Autodesk Inventor part; units mm, degrees
(part 2 of 3)
  spline S192 degree 2 poles (69.3995, 110.7069) (69.4696, 110.764) (69.7263, 110.8625) (69.8923, 110.8625) knots 0 0 0 1 2 2 2
  spline S193 degree 2 poles (69.8923, 110.8625) (70.0453, 110.8625) (70.2632, 110.7614) (70.4006, 110.5669) (70.4655, 110.2945) (70.4655, 110.126) knots 0 0 0 1 2 3 4 4 4
  line L261 (70.4655, 110.126) -> (70.4655, 108.6191)
  line L262 (70.4655, 108.6191) -> (70.0842, 108.6191)
  line L263 (70.0842, 108.6191) -> (70.0842, 110.1052)
  spline S194 degree 2 poles (70.0842, 110.1052) (70.0842, 110.2141) (70.0531, 110.3775) (69.9805, 110.4865) (69.856, 110.5409) (69.7626, 110.5409) knots 0 0 0 1 2 3 4 4 4
  spline S195 degree 2 poles (69.7626, 110.5409) (69.7056, 110.5409) (69.5785, 110.502) (69.4488, 110.4346) (69.3269, 110.349) (69.2725, 110.3049) knots 0 0 0 1 2 3 4 4 4
  spline S196 degree 2 poles (69.2725, 110.3049) (69.2776, 110.2453) (69.2802, 110.1675) (69.2802, 110.1052) knots 0 0 0 1 2 2 2
  line L264 (69.2802, 110.1052) -> (69.2802, 108.6191)
  line L265 (69.2802, 108.6191) -> (68.899, 108.6191)
  line L266 (68.899, 108.6191) -> (68.899, 110.1052)
  spline S197 degree 2 poles (68.899, 110.1052) (68.899, 110.3231) (68.7538, 110.5409) (68.567, 110.5409) knots 0 0 0 1 2 2 2
  spline S198 degree 2 poles (68.567, 110.5409) (68.5074, 110.5409) (68.3699, 110.5046) (68.2376, 110.4398) (68.108, 110.3594) (68.0561, 110.3153) knots 0 0 0 1 2 3 4 4 4
  line L267 (68.0561, 110.3153) -> (68.0561, 108.6191)
  spline S199 degree 2 poles (73.6192, 110.4657) (73.5829, 110.4839) (73.4818, 110.5202) (73.3728, 110.5487) (73.2639, 110.5643) (73.2146, 110.5643) knots 0 0 0 1 2 3 4 4 4
  spline S200 degree 2 poles (73.2146, 110.5643) (73.002, 110.5643) (72.8256, 110.4372) (72.8256, 110.3101) knots 0 0 0 1 2 2 2
  spline S201 degree 2 poles (72.8256, 110.3101) (72.8256, 110.2271) (72.9423, 110.1156) (73.1265, 110.0274) (73.3521, 109.9496) (73.461, 109.8951) knots 0 0 0 1 2 3 4 4 4
  spline S202 degree 2 poles (73.461, 109.8951) (73.5388, 109.8562) (73.6996, 109.7525) (73.8267, 109.6124) (73.9071, 109.4361) (73.9071, 109.3246) knots 0 0 0 1 2 3 4 4 4
  spline S203 degree 2 poles (73.9071, 109.3246) (73.9071, 109.1223) (73.7697, 108.8396) (73.5362, 108.6658) (73.2224, 108.5854) (73.0435, 108.5854) knots 0 0 0 1 2 3 4 4 4
  spline S204 degree 2 poles (73.0435, 108.5854) (72.9734, 108.5854) (72.8023, 108.6113) (72.6285, 108.658) (72.4729, 108.7229) (72.421, 108.7592) knots 0 0 0 1 2 3 4 4 4
  line L268 (72.421, 108.7592) -> (72.5533, 109.0237)
  spline S205 degree 2 poles (72.5533, 109.0237) (72.6026, 109.0004) (72.7348, 108.9563) (72.8749, 108.9252) (73.0123, 108.907) (73.0668, 108.907) knots 0 0 0 1 2 3 4 4 4
  spline S206 degree 2 poles (73.0668, 108.907) (73.1602, 108.907) (73.3313, 108.9459) (73.461, 109.0289) (73.5388, 109.1638) (73.5388, 109.2623) knots 0 0 0 1 2 3 4 4 4
  spline S207 degree 2 poles (73.5388, 109.2623) (73.5388, 109.3375) (73.4766, 109.449) (73.3703, 109.5346) (73.2302, 109.6073) (73.072, 109.6747) (72.9086, 109.7447) (72.8334, 109.7862) knots 0 0 0 1 2 3 4 5 6 6 6
  spline S208 degree 2 poles (72.8334, 109.7862) (72.7634, 109.8277) (72.6337, 109.9237) (72.5325, 110.043) (72.4729, 110.1934) (72.4729, 110.2894) knots 0 0 0 1 2 3 4 4 4
  spline S209 degree 2 poles (72.4729, 110.2894) (72.4729, 110.4424) (72.5818, 110.6628) (72.7789, 110.7977) (73.0538, 110.8625) (73.2198, 110.8625) knots 0 0 0 1 2 3 4 4 4
  spline S210 degree 2 poles (73.2198, 110.8625) (73.2976, 110.8625) (73.4455, 110.8392) (73.5829, 110.8003) (73.6944, 110.7484) (73.7333, 110.7225) knots 0 0 0 1 2 3 4 4 4
  line L269 (73.7333, 110.7225) -> (73.6192, 110.4657)
  line L270 (75.7252, 110.8288) -> (76.1064, 110.8677)
  line L271 (76.1064, 110.8677) -> (76.1064, 108.6191)
  line L272 (76.1064, 108.6191) -> (75.7252, 108.6191)
  line L273 (75.7252, 108.6191) -> (75.7252, 108.9459)
  line L274 (75.7252, 108.9459) -> (75.6033, 108.7332)
  spline S211 degree 2 poles (75.6033, 108.7332) (75.567, 108.7073) (75.4684, 108.6554) (75.3439, 108.6139) (75.1961, 108.5854) (75.1131, 108.5854) knots 0 0 0 1 2 3 4 4 4
  spline S212 degree 2 poles (75.1131, 108.5854) (74.9523, 108.5854) (74.7215, 108.7021) (74.5737, 108.9096) (74.501, 109.1975) (74.501, 109.3661) knots 0 0 0 1 2 3 4 4 4
  line L275 (74.501, 109.3661) -> (74.501, 110.8288)
  line L276 (74.501, 110.8288) -> (74.8823, 110.8677)
  line L277 (74.8823, 110.8677) -> (74.8823, 109.3661)
  spline S213 degree 2 poles (74.8823, 109.3661) (74.8823, 109.1508) (75.056, 108.907) (75.2428, 108.907) knots 0 0 0 1 2 2 2
  spline S214 degree 2 poles (75.2428, 108.907) (75.3128, 108.907) (75.4451, 108.9511) (75.5696, 109.0185) (75.6785, 109.0989) (75.7252, 109.1378) knots 0 0 0 1 2 3 4 4 4
  line L278 (75.7252, 109.1378) -> (75.7252, 110.8288)
  spline S215 degree 2 poles (77.8571, 110.5228) (77.7767, 110.5228) (77.6185, 110.4579) (77.4732, 110.349) (77.3461, 110.2064) (77.2917, 110.126) knots 0 0 0 1 2 3 4 4 4
  line L279 (77.2917, 110.126) -> (77.2917, 108.6191)
  line L280 (77.2917, 108.6191) -> (76.9104, 108.6191)
  line L281 (76.9104, 108.6191) -> (76.9104, 110.8288)
  line L282 (76.9104, 110.8288) -> (77.2917, 110.8677)
  line L283 (77.2917, 110.8677) -> (77.2917, 110.4164)
  line L284 (77.2917, 110.4164) -> (77.4914, 110.7692)
  spline S216 degree 2 poles (77.4914, 110.7692) (77.5173, 110.7847) (77.5977, 110.8184) (77.6963, 110.8444) (77.8104, 110.8625) (77.8726, 110.8625) knots 0 0 0 1 2 3 4 4 4
  spline S217 degree 2 poles (77.8726, 110.8625) (77.9634, 110.8625) (78.0853, 110.8314) (78.1138, 110.8158) knots 0 0 0 1 2 2 2
  line L285 (78.1138, 110.8158) -> (78.0957, 110.4839)
  spline S218 degree 2 poles (78.0957, 110.4839) (78.0646, 110.4916) (77.9453, 110.5228) (77.8571, 110.5228) knots 0 0 0 1 2 2 2
  line L286 (78.215, 110.8262) -> (78.5158, 110.8262)
  line L287 (78.5158, 110.8262) -> (78.5158, 111.1374)
  spline S219 degree 2 poles (78.5158, 111.1374) (78.5158, 111.3086) (78.591, 111.5757) (78.7492, 111.7625) (79.0008, 111.8636) (79.1772, 111.8636) knots 0 0 0 1 2 3 4 4 4
  spline S220 degree 2 poles (79.1772, 111.8636) (79.268, 111.8636) (79.4184, 111.8325) (79.5455, 111.7858) (79.6518, 111.721) (79.6933, 111.6873) knots 0 0 0 1 2 3 4 4 4
  line L288 (79.6933, 111.6873) -> (79.5221, 111.4487)
  spline S221 degree 2 poles (79.5221, 111.4487) (79.4806, 111.4798) (79.3328, 111.542) (79.242, 111.542) knots 0 0 0 1 2 2 2
  spline S222 degree 2 poles (79.242, 111.542) (79.0683, 111.542) (78.8867, 111.3475) (78.8867, 111.1167) knots 0 0 0 1 2 2 2
  line L289 (78.8867, 111.1167) -> (78.8867, 110.8262)
  line L290 (78.8867, 110.8262) -> (79.4703, 110.8262)
  line L291 (79.4703, 110.8262) -> (79.4288, 110.5046)
  line L292 (79.4288, 110.5046) -> (78.8971, 110.5046)
  line L293 (78.8971, 110.5046) -> (78.8971, 108.6191)
  line L294 (78.8971, 108.6191) -> (78.5158, 108.6191)
  line L295 (78.5158, 108.6191) -> (78.5158, 110.5046)
  line L296 (78.5158, 110.5046) -> (78.215, 110.5046)
  line L297 (78.215, 110.5046) -> (78.215, 110.8262)
  line L298 (81.5658, 108.6191) -> (81.1457, 108.6191)
  line L299 (81.1457, 108.6191) -> (81.1457, 108.9433)
  line L300 (81.1457, 108.9433) -> (80.9563, 108.7203)
  spline S223 degree 2 poles (80.9563, 108.7203) (80.9226, 108.6943) (80.8345, 108.6451) (80.7437, 108.6061) (80.6529, 108.5854) (80.614, 108.5854) knots 0 0 0 1 2 3 4 4 4
  spline S224 degree 2 poles (80.614, 108.5854) (80.4636, 108.5854) (80.1887, 108.6788) (79.9812, 108.8629) (79.8593, 109.1326) (79.8593, 109.3116) knots 0 0 0 1 2 3 4 4 4
  spline S225 degree 2 poles (79.8593, 109.3116) (79.8593, 109.4983) (80.0097, 109.7732) (80.2457, 109.9548) (80.5336, 110.0456) (80.6737, 110.0456) knots 0 0 0 1 2 3 4 4 4
  spline S226 degree 2 poles (80.6737, 110.0456) (80.7878, 110.0456) (80.9615, 110.0222) (81.0238, 110.0067) knots 0 0 0 1 2 2 2
  spline S227 degree 2 poles (81.0238, 110.0067) (81.0938, 109.9885) (81.1457, 109.9652) knots 0 0 0 1 1 1
  line L301 (81.1457, 109.9652) -> (81.1457, 110.0352)
  spline S228 degree 2 poles (81.1457, 110.0352) (81.1457, 110.1545) (81.1171, 110.3412) (81.0316, 110.4735) (80.8682, 110.5409) (80.7333, 110.5409) knots 0 0 0 1 2 3 4 4 4
  spline S229 degree 2 poles (80.7333, 110.5409) (80.6244, 110.5409) (80.4247, 110.5098) (80.3469, 110.4916) knots 0 0 0 1 2 2 2
  spline S230 degree 2 poles (80.3469, 110.4916) (80.2535, 110.4709) (80.1757, 110.4476) knots 0 0 0 1 1 1
  line L302 (80.1757, 110.4476) -> (80.0305, 110.7147)
  spline S231 degree 2 poles (80.0305, 110.7147) (80.1186, 110.7562) (80.2302, 110.7873) knots 0 0 0 1 1 1
  spline S232 degree 2 poles (80.2302, 110.7873) (80.3261, 110.8158) (80.5933, 110.8625) (80.7541, 110.8625) knots 0 0 0 1 2 2 2
  spline S233 degree 2 poles (80.7541, 110.8625) (80.9849, 110.8625) (81.2857, 110.738) (81.4595, 110.5124) (81.5269, 110.1986) (81.5269, 110.0041) knots 0 0 0 1 2 3 4 4 4
  line L303 (81.5269, 110.0041) -> (81.5269, 108.9796)
  line L304 (81.5269, 108.9796) -> (81.5658, 108.6191)
  spline S234 degree 2 poles (81.1457, 109.6902) (81.0886, 109.698) (81.0238, 109.7058) knots 0 0 0 1 1 1
  spline S235 degree 2 poles (81.0238, 109.7058) (80.9719, 109.711) (80.8293, 109.724) (80.7541, 109.724) knots 0 0 0 1 2 2 2
  spline S236 degree 2 poles (80.7541, 109.724) (80.6399, 109.724) (80.4532, 109.6799) (80.3157, 109.5813) (80.2405, 109.4257) (80.2405, 109.3116) knots 0 0 0 1 2 3 4 4 4
  spline S237 degree 2 poles (80.2405, 109.3116) (80.2405, 109.2234) (80.3002, 109.073) (80.4065, 108.9641) (80.5492, 108.907) (80.6296, 108.907) knots 0 0 0 1 2 3 4 4 4
  spline S238 degree 2 poles (80.6296, 108.907) (80.6685, 108.907) (80.7566, 108.9303) (80.8422, 108.9641) (80.9278, 109.0133) (80.9667, 109.0367) knots 0 0 0 1 2 3 4 4 4
  spline S239 degree 2 poles (80.9667, 109.0367) (81.0575, 109.0963) (81.1457, 109.1689) knots 0 0 0 1 1 1
  line L305 (81.1457, 109.1689) -> (81.1457, 109.6902)
  spline S240 degree 2 poles (83.4461, 110.3827) (83.3683, 110.4527) (83.1531, 110.5409) (83.039, 110.5409) knots 0 0 0 1 2 2 2
  spline S241 degree 2 poles (83.039, 110.5409) (82.8704, 110.5409) (82.6344, 110.4138) (82.4865, 110.1986) (82.4191, 109.9107) (82.4191, 109.7525) knots 0 0 0 1 2 3 4 4 4
  spline S242 degree 2 poles (82.4191, 109.7525) (82.4191, 109.5865) (82.4813, 109.2882) (82.6292, 109.06) (82.8756, 108.9252) (83.0623, 108.9252) knots 0 0 0 1 2 3 4 4 4
  spline S243 degree 2 poles (83.0623, 108.9252) (83.2153, 108.9252) (83.4306, 108.9978) (83.4902, 109.0367) knots 0 0 0 1 2 2 2
  line L306 (83.4902, 109.0367) -> (83.6329, 108.754)
  spline S244 degree 2 poles (83.6329, 108.754) (83.5214, 108.6788) (83.2231, 108.5854) (83.0338, 108.5854) knots 0 0 0 1 2 2 2
  spline S245 degree 2 poles (83.0338, 108.5854) (82.7822, 108.5854) (82.4061, 108.7851) (82.1546, 109.1145) (82.0275, 109.5476) (82.0275, 109.7784) knots 0 0 0 1 2 3 4 4 4
  spline S246 degree 2 poles (82.0275, 109.7784) (82.0275, 109.9859) (82.1494, 110.3775) (82.4009, 110.681) (82.7848, 110.8625) (83.0441, 110.8625) knots 0 0 0 1 2 3 4 4 4
  spline S247 degree 2 poles (83.0441, 110.8625) (83.2283, 110.8625) (83.5188, 110.7484) (83.6458, 110.6084) knots 0 0 0 1 2 2 2
  line L307 (83.6458, 110.6084) -> (83.4461, 110.3827)
  spline S248 degree 2 poles (85.7725, 108.8785) (85.7103, 108.8136) (85.5625, 108.7073) (85.3809, 108.6269) (85.1631, 108.5854) (85.0282, 108.5854) knots 0 0 0 1 2 3 4 4 4
  spline S249 degree 2 poles (85.0282, 108.5854) (84.7611, 108.5854) (84.385, 108.7747) (84.1464, 109.0911) (84.0349, 109.5009) (84.0349, 109.724) knots 0 0 0 1 2 3 4 4 4
  spline S250 degree 2 poles (84.0349, 109.724) (84.0349, 109.8666) (84.0867, 110.1467) (84.1905, 110.3983) (84.3487, 110.6161) (84.5562, 110.7718) (84.8207, 110.8625) (84.9789, 110.8625) knots 0 0 0 1 2 3 4 5 6 6 6
  spline S251 degree 2 poles (84.9789, 110.8625) (85.1942, 110.8625) (85.5132, 110.7225) (85.7207, 110.4683) (85.8218, 110.1156) (85.8218, 109.9003) knots 0 0 0 1 2 3 4 4 4
  spline S252 degree 2 poles (85.8218, 109.9003) (85.8218, 109.8381) (85.814, 109.6902) (85.8063, 109.6228) knots 0 0 0 1 2 2 2
  line L308 (85.8063, 109.6228) -> (84.4161, 109.6228)
  spline S253 degree 2 poles (84.4161, 109.6228) (84.4161, 109.4724) (84.4991, 109.213) (84.647, 109.0185) (84.857, 108.907) (84.9893, 108.907) knots 0 0 0 1 2 3 4 4 4
  spline S254 degree 2 poles (84.9893, 108.907) (85.1164, 108.907) (85.3083, 108.9459) (85.4432, 109.0004) (85.5313, 109.0548) (85.5547, 109.0704) knots 0 0 0 1 2 3 4 4 4
  line L309 (85.5547, 109.0704) -> (85.7725, 108.8785)
  spline S255 degree 2 poles (85.4406, 109.9237) (85.4432, 109.947) (85.4458, 109.9911) (85.4458, 110.0118) knots 0 0 0 1 2 2 2
  spline S256 degree 2 poles (85.4458, 110.0118) (85.4458, 110.126) (85.3913, 110.3205) (85.285, 110.4631) (85.1216, 110.5435) (85.0075, 110.5435) knots 0 0 0 1 2 3 4 4 4
  spline S257 degree 2 poles (85.0075, 110.5435) (84.8752, 110.5435) (84.6833, 110.4579) (84.5536, 110.3231) (84.4732, 110.1623) (84.455, 110.0897) knots 0 0 0 1 2 3 4 4 4
  line L310 (84.455, 110.0897) -> (84.3487, 109.8692)
  line L311 (84.3487, 109.8692) -> (84.7066, 109.9237)
  line L312 (84.7066, 109.9237) -> (85.4406, 109.9237)
  spline S258 degree 2 poles (87.4454, 108.6191) (87.4454, 108.4402) (87.4091, 108.1315) (87.2872, 107.9033) (87.0486, 107.7762) (86.8437, 107.7762) knots 0 0 0 1 2 3 4 4 4
  spline S259 degree 2 poles (86.8437, 107.7762) (86.8048, 107.7762) (86.7218, 107.7814) (86.644, 107.7944) (86.5817, 107.8151) (86.5636, 107.8255) knots 0 0 0 1 2 3 4 4 4
  line L313 (86.5636, 107.8255) -> (86.7036, 108.0797)
  spline S260 degree 2 poles (86.7036, 108.0797) (86.714, 108.0745) (86.7296, 108.0719) knots 0 0 0 1 1 1
  spline S261 degree 2 poles (86.7296, 108.0719) (86.7451, 108.0719) (86.7814, 108.0693) (86.8022, 108.0693) knots 0 0 0 1 2 2 2
  spline S262 degree 2 poles (86.8022, 108.0693) (86.8904, 108.0693) (86.9889, 108.1523) (87.0356, 108.2975) (87.0434, 108.4868) (87.0434, 108.5906) knots 0 0 0 1 2 3 4 4 4
  line L314 (87.0434, 108.5906) -> (87.0434, 111.0155)
  spline S263 degree 2 poles (87.0434, 111.0155) (87.0434, 111.1193) (87.0356, 111.3086) (86.9889, 111.4539) (86.8904, 111.5368) (86.8022, 111.5368) knots 0 0 0 1 2 3 4 4 4
  spline S264 degree 2 poles (86.8022, 111.5368) (86.7814, 111.5368) (86.7451, 111.5343) (86.7296, 111.5317) knots 0 0 0 1 2 2 2
  spline S265 degree 2 poles (86.7296, 111.5317) (86.714, 111.5291) (86.7036, 111.5291) knots 0 0 0 1 1 1
  line L315 (86.7036, 111.5291) -> (86.5636, 111.7806)
  spline S266 degree 2 poles (86.5636, 111.7806) (86.5817, 111.7936) (86.644, 111.8118) (86.7218, 111.8247) (86.8048, 111.8299) (86.8437, 111.8299) knots 0 0 0 1 2 3 4 4 4
  spline S267 degree 2 poles (86.8437, 111.8299) (87.0486, 111.8299) (87.2872, 111.7028) (87.4091, 111.4746) (87.4454, 111.166) (87.4454, 110.987) knots 0 0 0 1 2 3 4 4 4
  line L316 (87.4454, 110.987) -> (87.4454, 108.6191)
  line L317 (32.347, 101.896) -> (32.347, 102.2176)
  line L318 (32.347, 102.2176) -> (32.8397, 102.2176)
  line L319 (32.8397, 102.2176) -> (32.8397, 104.1549)
  line L320 (32.8397, 104.1549) -> (32.9565, 104.6114)
  line L321 (32.9565, 104.6114) -> (32.6841, 104.2379)
  line L322 (32.6841, 104.2379) -> (32.2588, 103.8619)
  line L323 (32.2588, 103.8619) -> (32.0409, 104.1031)
  line L324 (32.0409, 104.1031) -> (32.9616, 104.946)
  line L325 (32.9616, 104.946) -> (33.2625, 104.9071)
  line L326 (33.2625, 104.9071) -> (33.2625, 102.2176)
  line L327 (33.2625, 102.2176) -> (33.7553, 102.2176)
  line L328 (33.7553, 102.2176) -> (33.7553, 101.896)
  line L329 (33.7553, 101.896) -> (32.347, 101.896)
  line L330 (34.829, 101.6963) -> (34.4062, 101.6963)
  line L331 (34.4062, 101.6963) -> (35.8327, 105.1068)
  line L332 (35.8327, 105.1068) -> (36.2321, 105.1068)
  line L333 (36.2321, 105.1068) -> (34.829, 101.6963)
  line L334 (38.6415, 102.4977) -> (38.281, 102.4977)
  line L335 (38.281, 102.4977) -> (38.281, 101.896)
  line L336 (38.281, 101.896) -> (37.8582, 101.896)
  line L337 (37.8582, 101.896) -> (37.8582, 102.4977)
  line L338 (37.8582, 102.4977) -> (36.6626, 102.4977)
  line L339 (36.6626, 102.4977) -> (36.6626, 102.84)
  line L340 (36.6626, 102.84) -> (37.6352, 104.946)
  line L341 (37.6352, 104.946) -> (38.0164, 104.9071)
  line L342 (38.0164, 104.9071) -> (37.1813, 103.0994)
  line L343 (37.1813, 103.0994) -> (36.9946, 102.8193)
  line L344 (36.9946, 102.8193) -> (37.8582, 102.8193)
  line L345 (37.8582, 102.8193) -> (37.8582, 103.6362)
  line L346 (37.8582, 103.6362) -> (38.281, 103.6025)
  line L347 (38.281, 103.6025) -> (38.281, 102.8193)
  line L348 (38.281, 102.8193) -> (38.6726, 102.8193)
  line L349 (38.6726, 102.8193) -> (38.6415, 102.4977)
  line L350 (40.3273, 104.9071) -> (40.3273, 104.7074)
  spline S268 degree 2 poles (40.3273, 104.7074) (40.3273, 104.6295) (40.2988, 104.4065) (40.2832, 104.2976) knots 0 0 0 1 2 2 2
  spline S269 degree 2 poles (40.2832, 104.2976) (40.2624, 104.1731) (40.2391, 104.0382) knots 0 0 0 1 1 1
  line L351 (40.2391, 104.0382) -> (40.0653, 104.0382)
  spline S270 degree 2 poles (40.0653, 104.0382) (40.042, 104.1731) (40.0212, 104.2976) knots 0 0 0 1 1 1
  spline S271 degree 2 poles (40.0212, 104.2976) (40.0057, 104.4065) (39.9772, 104.6295) (39.9772, 104.7074) knots 0 0 0 1 2 2 2
  line L352 (39.9772, 104.7074) -> (39.9772, 104.9071)
  line L353 (39.9772, 104.9071) -> (40.3273, 104.9071)
  line L354 (39.723, 104.9071) -> (39.723, 104.7074)
  spline S272 degree 2 poles (39.723, 104.7074) (39.723, 104.6295) (39.6945, 104.4065) (39.6789, 104.2976) knots 0 0 0 1 2 2 2
  spline S273 degree 2 poles (39.6789, 104.2976) (39.6582, 104.1731) (39.6348, 104.0382) knots 0 0 0 1 1 1
  line L355 (39.6348, 104.0382) -> (39.461, 104.0382)
  spline S274 degree 2 poles (39.461, 104.0382) (39.4377, 104.1731) (39.417, 104.2976) knots 0 0 0 1 1 1
  spline S275 degree 2 poles (39.417, 104.2976) (39.4014, 104.4065) (39.3729, 104.6295) (39.3729, 104.7074) knots 0 0 0 1 2 2 2
  line L356 (39.3729, 104.7074) -> (39.3729, 104.9071)
  line L357 (39.3729, 104.9071) -> (39.723, 104.9071)
  line L358 (42.4851, 104.7463) -> (42.4462, 105.1094)
  line L359 (42.4462, 105.1094) -> (42.8664, 105.1483)
  line L360 (42.8664, 105.1483) -> (42.8664, 103.8515)
  line L361 (42.8664, 103.8515) -> (43.0375, 104.0356)
  spline S276 degree 2 poles (43.0375, 104.0356) (43.1387, 104.0823) (43.3643, 104.1394) (43.4758, 104.1394) knots 0 0 0 1 2 2 2
  spline S277 degree 2 poles (43.4758, 104.1394) (43.6418, 104.1394) (43.9375, 104.0019) (44.1605, 103.7348) (44.2902, 103.3457) (44.2902, 103.0942) knots 0 0 0 1 2 3 4 4 4
  spline S278 degree 2 poles (44.2902, 103.0942) (44.2902, 102.8167) (44.1398, 102.3628) (43.8701, 102.0386) (43.4992, 101.8622) (43.2761, 101.8622) knots 0 0 0 1 2 3 4 4 4
  spline S279 degree 2 poles (43.2761, 101.8622) (43.1516, 101.8622) (42.9053, 101.8804) (42.6926, 101.9115) (42.5292, 101.9478) (42.4851, 101.966) knots 0 0 0 1 2 3 4 4 4
  line L362 (42.4851, 101.966) -> (42.4851, 104.7463)
  spline S280 degree 2 poles (42.8664, 102.2409) (42.9053, 102.2279) (43.0038, 102.2072) (43.1179, 102.1916) (43.2398, 102.1838) (43.2943, 102.1838) knots 0 0 0 1 2 3 4 4 4
  spline S281 degree 2 poles (43.2943, 102.1838) (43.4188, 102.1838) (43.6055, 102.2642) (43.7404, 102.3991) (43.8312, 102.5807) (43.8882, 102.7829) (43.909, 103.0008) (43.909, 103.102) knots 0 0 0 1 2 3 4 5 6 6 6
  spline S282 degree 2 poles (43.909, 103.102) (43.909, 103.3043) (43.8337, 103.5766) (43.7015, 103.7452) (43.5329, 103.8178) (43.4369, 103.8178) knots 0 0 0 1 2 3 4 4 4
  spline S283 degree 2 poles (43.4369, 103.8178) (43.2787, 103.8178) (42.9908, 103.6959) (42.8664, 103.5921) knots 0 0 0 1 2 2 2
  line L363 (42.8664, 103.5921) -> (42.8664, 102.2409)
  line L364 (45.2758, 101.896) -> (44.8945, 101.896)
  line L365 (44.8945, 101.896) -> (44.8945, 104.0149)
  line L366 (44.8945, 104.0149) -> (45.2758, 104.0564)
  line L367 (45.2758, 104.0564) -> (45.2758, 101.896)
  line L368 (44.8815, 104.9071) -> (45.2887, 104.9071)
  line L369 (45.2887, 104.9071) -> (45.2887, 104.5051)
  line L370 (45.2887, 104.5051) -> (44.8815, 104.5051)
  line L371 (44.8815, 104.5051) -> (44.8815, 104.9071)
  spline S284 degree 2 poles (46.4792, 102.6507) (46.4792, 102.5184) (46.5103, 102.3395) (46.5673, 102.2305) (46.6529, 102.1838) (46.71, 102.1838) knots 0 0 0 1 2 3 4 4 4
  spline S285 degree 2 poles (46.71, 102.1838) (46.7541, 102.1838) (46.8267, 102.1942) (46.8526, 102.202) knots 0 0 0 1 2 2 2
  spline S286 degree 2 poles (46.8526, 102.202) (46.8837, 102.2098) (46.9071, 102.2202) knots 0 0 0 1 1 1
  line L372 (46.9071, 102.2202) -> (47.0445, 101.9764)
  spline S287 degree 2 poles (47.0445, 101.9764) (47.029, 101.9608) (46.959, 101.9219) (46.863, 101.8856) (46.7411, 101.8622) (46.6711, 101.8622) knots 0 0 0 1 2 3 4 4 4
  spline S288 degree 2 poles (46.6711, 101.8622) (46.4895, 101.8622) (46.2639, 101.9945) (46.1394, 102.2227) (46.0979, 102.5262) (46.0979, 102.6974) knots 0 0 0 1 2 3 4 4 4
  line L373 (46.0979, 102.6974) -> (46.0979, 103.7815)
  line L374 (46.0979, 103.7815) -> (45.7971, 103.7815)
  line L375 (45.7971, 103.7815) -> (45.7971, 104.1031)
  line L376 (45.7971, 104.1031) -> (46.0979, 104.1031)
  line L377 (46.0979, 104.1031) -> (46.0979, 104.5232)
  line L378 (46.0979, 104.5232) -> (46.4688, 104.7463)
  line L379 (46.4688, 104.7463) -> (46.4688, 104.1031)
  line L380 (46.4688, 104.1031) -> (47.1509, 104.1031)
  line L381 (47.1509, 104.1031) -> (47.112, 103.7815)
  line L382 (47.112, 103.7815) -> (46.4792, 103.7815)
  line L383 (46.4792, 103.7815) -> (46.4792, 102.6507)
  spline S289 degree 2 poles (47.5062, 102.1631) (47.5062, 102.2202) (47.5529, 102.3265) (47.6333, 102.4043) (47.7422, 102.451) (47.8045, 102.451) knots 0 0 0 1 2 3 4 4 4
  spline S290 degree 2 poles (47.8045, 102.451) (47.8615, 102.451) (47.9678, 102.4095) (48.0508, 102.3291) (48.1001, 102.2072) (48.1001, 102.1294) knots 0 0 0 1 2 3 4 4 4
  spline S291 degree 2 poles (48.1001, 102.1294) (48.1001, 102.023) (48.0742, 101.8233) (47.9912, 101.6185) (47.8382, 101.4058) (47.7137, 101.2917) knots 0 0 0 1 2 3 4 4 4
  line L384 (47.7137, 101.2917) -> (47.6099, 101.3383)
  spline S292 degree 2 poles (47.6099, 101.3383) (47.6566, 101.4265) (47.6929, 101.5199) knots 0 0 0 1 1 1
  spline S293 degree 2 poles (47.6929, 101.5199) (47.7241, 101.5977) (47.7733, 101.7844) (47.7733, 101.8726) knots 0 0 0 1 2 2 2
  spline S294 degree 2 poles (47.7733, 101.8726) (47.7241, 101.8752) (47.6255, 101.9167) (47.5503, 101.9867) (47.5062, 102.0957) (47.5062, 102.1631) knots 0 0 0 1 2 3 4 4 4
  line L385 (51.3369, 104.1057) -> (51.7181, 104.1446)
  line L386 (51.7181, 104.1446) -> (51.7181, 101.896)
  line L387 (51.7181, 101.896) -> (51.3369, 101.896)
  line L388 (51.3369, 101.896) -> (51.3369, 102.2227)
  line L389 (51.3369, 102.2227) -> (51.215, 102.0101)
  spline S295 degree 2 poles (51.215, 102.0101) (51.1786, 101.9841) (51.0801, 101.9323) (50.9556, 101.8908) (50.8078, 101.8622) (50.7248, 101.8622) knots 0 0 0 1 2 3 4 4 4
  spline S296 degree 2 poles (50.7248, 101.8622) (50.564, 101.8622) (50.3332, 101.979) (50.1853, 102.1864) (50.1127, 102.4743) (50.1127, 102.6429) knots 0 0 0 1 2 3 4 4 4
  line L390 (50.1127, 102.6429) -> (50.1127, 104.1057)
  line L391 (50.1127, 104.1057) -> (50.494, 104.1446)
  line L392 (50.494, 104.1446) -> (50.494, 102.6429)
  spline S297 degree 2 poles (50.494, 102.6429) (50.494, 102.4276) (50.6677, 102.1838) (50.8545, 102.1838) knots 0 0 0 1 2 2 2
  spline S298 degree 2 poles (50.8545, 102.1838) (50.9245, 102.1838) (51.0568, 102.2279) (51.1812, 102.2954) (51.2902, 102.3758) (51.3369, 102.4147) knots 0 0 0 1 2 3 4 4 4
  line L393 (51.3369, 102.4147) -> (51.3369, 104.1057)
  spline S299 degree 2 poles (53.448, 103.7426) (53.4117, 103.7607) (53.3105, 103.797) (53.2016, 103.8256) (53.0927, 103.8411) (53.0434, 103.8411) knots 0 0 0 1 2 3 4 4 4
  spline S300 degree 2 poles (53.0434, 103.8411) (52.8307, 103.8411) (52.6544, 103.714) (52.6544, 103.5869) knots 0 0 0 1 2 2 2
  spline S301 degree 2 poles (52.6544, 103.5869) (52.6544, 103.504) (52.7711, 103.3924) (52.9552, 103.3043) (53.1809, 103.2264) (53.2898, 103.172) knots 0 0 0 1 2 3 4 4 4
  spline S302 degree 2 poles (53.2898, 103.172) (53.3676, 103.1331) (53.5284, 103.0293) (53.6555, 102.8893) (53.7359, 102.7129) (53.7359, 102.6014) knots 0 0 0 1 2 3 4 4 4
  spline S303 degree 2 poles (53.7359, 102.6014) (53.7359, 102.3991) (53.5984, 102.1164) (53.365, 101.9426) (53.0512, 101.8622) (52.8722, 101.8622) knots 0 0 0 1 2 3 4 4 4
  spline S304 degree 2 poles (52.8722, 101.8622) (52.8022, 101.8622) (52.631, 101.8882) (52.4573, 101.9349) (52.3016, 101.9997) (52.2498, 102.036) knots 0 0 0 1 2 3 4 4 4
  line L394 (52.2498, 102.036) -> (52.382, 102.3006)
  spline S305 degree 2 poles (52.382, 102.3006) (52.4313, 102.2772) (52.5636, 102.2331) (52.7036, 102.202) (52.8411, 102.1838) (52.8956, 102.1838) knots 0 0 0 1 2 3 4 4 4
  spline S306 degree 2 poles (52.8956, 102.1838) (52.9889, 102.1838) (53.1601, 102.2227) (53.2898, 102.3057) (53.3676, 102.4406) (53.3676, 102.5392) knots 0 0 0 1 2 3 4 4 4
  spline S307 degree 2 poles (53.3676, 102.5392) (53.3676, 102.6144) (53.3053, 102.7259) (53.199, 102.8115) (53.059, 102.8841) (52.9008, 102.9515) (52.7374, 103.0216) (52.6622, 103.0631) knots 0 0 0 1 2 3 4 5 6 6 6
  spline S308 degree 2 poles (52.6622, 103.0631) (52.5921, 103.1045) (52.4624, 103.2005) (52.3613, 103.3198) (52.3016, 103.4702) (52.3016, 103.5662) knots 0 0 0 1 2 3 4 4 4
  spline S309 degree 2 poles (52.3016, 103.5662) (52.3016, 103.7192) (52.4106, 103.9397) (52.6077, 104.0745) (52.8826, 104.1394) (53.0486, 104.1394) knots 0 0 0 1 2 3 4 4 4
  spline S310 degree 2 poles (53.0486, 104.1394) (53.1264, 104.1394) (53.2742, 104.116) (53.4117, 104.0771) (53.5232, 104.0253) (53.5621, 103.9993) knots 0 0 0 1 2 3 4 4 4
  line L395 (53.5621, 103.9993) -> (53.448, 103.7426)
  spline S311 degree 2 poles (55.8652, 102.1553) (55.8029, 102.0905) (55.6551, 101.9841) (55.4735, 101.9037) (55.2557, 101.8622) (55.1208, 101.8622) knots 0 0 0 1 2 3 4 4 4
  spline S312 degree 2 poles (55.1208, 101.8622) (54.8537, 101.8622) (54.4776, 102.0516) (54.239, 102.368) (54.1275, 102.7778) (54.1275, 103.0008) knots 0 0 0 1 2 3 4 4 4
  spline S313 degree 2 poles (54.1275, 103.0008) (54.1275, 103.1435) (54.1794, 103.4236) (54.2831, 103.6751) (54.4413, 103.893) (54.6488, 104.0486) (54.9133, 104.1394) (55.0715, 104.1394) knots 0 0 0 1 2 3 4 5 6 6 6
  spline S314 degree 2 poles (55.0715, 104.1394) (55.2868, 104.1394) (55.6058, 103.9993) (55.8133, 103.7452) (55.9144, 103.3924) (55.9144, 103.1772) knots 0 0 0 1 2 3 4 4 4
  spline S315 degree 2 poles (55.9144, 103.1772) (55.9144, 103.1149) (55.9067, 102.9671) (55.8989, 102.8997) knots 0 0 0 1 2 2 2
  line L396 (55.8989, 102.8997) -> (54.5087, 102.8997)
  spline S316 degree 2 poles (54.5087, 102.8997) (54.5087, 102.7492) (54.5917, 102.4899) (54.7396, 102.2954) (54.9497, 102.1838) (55.0819, 102.1838) knots 0 0 0 1 2 3 4 4 4
  spline S317 degree 2 poles (55.0819, 102.1838) (55.209, 102.1838) (55.4009, 102.2227) (55.5358, 102.2772) (55.624, 102.3317) (55.6473, 102.3472) knots 0 0 0 1 2 3 4 4 4
  line L397 (55.6473, 102.3472) -> (55.8652, 102.1553)
  spline S318 degree 2 poles (55.5332, 103.2005) (55.5358, 103.2239) (55.5384, 103.2679) (55.5384, 103.2887) knots 0 0 0 1 2 2 2
  spline S319 degree 2 poles (55.5384, 103.2887) (55.5384, 103.4028) (55.4839, 103.5973) (55.3776, 103.74) (55.2142, 103.8204) (55.1001, 103.8204) knots 0 0 0 1 2 3 4 4 4
  spline S320 degree 2 poles (55.1001, 103.8204) (54.9678, 103.8204) (54.7759, 103.7348) (54.6462, 103.5999) (54.5658, 103.4391) (54.5477, 103.3665) knots 0 0 0 1 2 3 4 4 4
  line L398 (54.5477, 103.3665) -> (54.4413, 103.146)
  line L399 (54.4413, 103.146) -> (54.7992, 103.2005)
  line L400 (54.7992, 103.2005) -> (55.5332, 103.2005)
  spline S321 degree 2 poles (58.7466, 101.8622) (58.5754, 101.8622) (58.2901, 101.9919) (58.0645, 102.2176) (57.8933, 102.5184) (57.7792, 102.8608) (57.7221, 103.2239) (57.7221, 103.4028) knots 0 0 0 1 2 3 4 5 6 6 6
  spline S322 degree 2 poles (57.7221, 103.4028) (57.7221, 103.5818) (57.7714, 103.9526) (57.8752, 104.2924) (58.0386, 104.5906) (58.2642, 104.8111) (58.5599, 104.9408) (58.7466, 104.9408) knots 0 0 0 1 2 3 4 5 6 6 6
  spline S323 degree 2 poles (58.7466, 104.9408) (58.9178, 104.9408) (59.2031, 104.8111) (59.4287, 104.5855) (59.5999, 104.2846) (59.714, 103.9423) (59.771, 103.5766) (59.771, 103.4028) knots 0 0 0 1 2 3 4 5 6 6 6
  spline S324 degree 2 poles (59.771, 103.4028) (59.771, 103.2213) (59.7218, 102.8504) (59.618, 102.5106) (59.4546, 102.2124) (59.229, 101.9919) (58.9307, 101.8622) (58.7466, 101.8622) knots 0 0 0 1 2 3 4 5 6 6 6
  spline S325 degree 2 poles (58.1397, 103.4884) (58.1397, 103.3717) (58.1553, 103.0916) (58.2045, 102.8089) (58.2901, 102.5443) (58.4276, 102.3369) (58.6273, 102.2124) (58.7622, 102.2124) knots 0 0 0 1 2 3 4 5 6 6 6
  spline S326 degree 2 poles (58.7622, 102.2124) (58.884, 102.2124) (59.0682, 102.3057) (59.2005, 102.4691) (59.2835, 102.6844) (59.3327, 102.9282) (59.3535, 103.1901) (59.3535, 103.3146) knots 0 0 0 1 2 3 4 5 6 6 6
  spline S327 degree 2 poles (59.3535, 103.3146) (59.3535, 103.4313) (59.3379, 103.7114) (59.2886, 103.9915) (59.2031, 104.2587) (59.0656, 104.4636) (58.8659, 104.5881) (58.731, 104.5881) knots 0 0 0 1 2 3 4 5 6 6 6
  spline S328 degree 2 poles (58.731, 104.5881) (58.6091, 104.5881) (58.425, 104.4947) (58.2927, 104.3339) (58.2097, 104.116) (58.1604, 103.8722) (58.1397, 103.6129) (58.1397, 103.4884) knots 0 0 0 1 2 3 4 5 6 6 6
  spline S329 degree 2 poles (60.3235, 102.1968) (60.3235, 102.2642) (60.3753, 102.3861) (60.4661, 102.4769) (60.5828, 102.5288) (60.6528, 102.5288) knots 0 0 0 1 2 3 4 4 4
  spline S330 degree 2 poles (60.6528, 102.5288) (60.7203, 102.5288) (60.8396, 102.4769) (60.9303, 102.3861) (60.9822, 102.2642) (60.9822, 102.1968) knots 0 0 0 1 2 3 4 4 4
  spline S331 degree 2 poles (60.9822, 102.1968) (60.9822, 102.1294) (60.9303, 102.0075) (60.8422, 101.9167) (60.7229, 101.8622) (60.6554, 101.8622) knots 0 0 0 1 2 3 4 4 4
  spline S332 degree 2 poles (60.6554, 101.8622) (60.588, 101.8622) (60.4661, 101.9167) (60.3753, 102.0075) (60.3235, 102.1294) (60.3235, 102.1968) knots 0 0 0 1 2 3 4 4 4
  line L401 (61.7862, 104.5855) -> (61.8147, 104.9071)
  line L402 (61.8147, 104.9071) -> (63.2801, 104.9071)
  line L403 (63.2801, 104.9071) -> (63.2801, 104.627)
  spline S333 degree 2 poles (63.2801, 104.627) (63.2568, 104.5466) (63.1426, 104.3702) (62.987, 104.1938) (62.8055, 104.0201) (62.7121, 103.9423) knots 0 0 0 1 2 3 4 4 4
  line L404 (62.7121, 103.9423) -> (62.4476, 103.7944)
  spline S334 degree 2 poles (62.4476, 103.7944) (62.4683, 103.797) (62.5306, 103.7996) (62.5591, 103.7996) knots 0 0 0 1 2 2 2
  spline S335 degree 2 poles (62.5591, 103.7996) (62.7536, 103.7996) (63.0882, 103.7037) (63.3346, 103.5091) (63.4772, 103.2083) (63.4772, 103.006) knots 0 0 0 1 2 3 4 4 4
  spline S336 degree 2 poles (63.4772, 103.006) (63.4772, 102.8115) (63.332, 102.4951) (63.083, 102.2487) (62.7458, 102.0697) (62.362, 101.953) (61.9522, 101.896) (61.7551, 101.896) knots 0 0 0 1 2 3 4 5 6 6 6
  line L405 (61.7551, 101.896) -> (61.7551, 102.2176)
  spline S337 degree 2 poles (61.7551, 102.2176) (61.9211, 102.2227) (62.2427, 102.272) (62.5306, 102.3576) (62.7769, 102.4821) (62.9533, 102.6507) (63.0545, 102.8582) (63.0545, 102.9878) knots 0 0 0 1 2 3 4 5 6 6 6
  spline S338 degree 2 poles (63.0545, 102.9878) (63.0545, 103.1305) (62.9326, 103.325) (62.7199, 103.4365) (62.432, 103.4832) (62.2686, 103.4832) knots 0 0 0 1 2 3 4 4 4
  spline S339 degree 2 poles (62.2686, 103.4832) (62.2038, 103.4832) (62.0533, 103.478) (61.9937, 103.4728) knots 0 0 0 1 2 2 2
  line L406 (61.9937, 103.4728) -> (61.9937, 103.7841)
  spline S340 degree 2 poles (61.9937, 103.7841) (62.0767, 103.8437) (62.2686, 103.9967) (62.4657, 104.1627) (62.6525, 104.3339) (62.8055, 104.4869) (62.9092, 104.6192) (62.9248, 104.6659) knots 0 0 0 1 2 3 4 5 6 6 6
  line L407 (62.9248, 104.6659) -> (62.6213, 104.5855)
  line L408 (62.6213, 104.5855) -> (61.7862, 104.5855)
  spline S341 degree 2 poles (65.6636, 103.2264) (65.5443, 103.1331) (65.3056, 103.0449) (65.1552, 103.0449) knots 0 0 0 1 2 2 2
  spline S342 degree 2 poles (65.1552, 103.0449) (64.9607, 103.0449) (64.6184, 103.1746) (64.3668, 103.4158) (64.2215, 103.7555) (64.2215, 103.9656) knots 0 0 0 1 2 3 4 4 4
  spline S343 degree 2 poles (64.2215, 103.9656) (64.2215, 104.1809) (64.359, 104.5388) (64.6158, 104.7981) (64.9789, 104.9408) (65.2019, 104.9408) knots 0 0 0 1 2 3 4 4 4
  spline S344 degree 2 poles (65.2019, 104.9408) (65.4042, 104.9408) (65.7102, 104.8163) (65.9359, 104.6114) (66.0863, 104.3469) (66.1745, 104.0616) (66.2134, 103.7815) (66.2134, 103.6622) knots 0 0 0 1 2 3 4 5 6 6 6
  spline S345 degree 2 poles (66.2134, 103.6622) (66.2134, 103.4287) (66.12, 102.9852) (65.9359, 102.5936) (65.6713, 102.2616) (65.3342, 102.0179) (64.9218, 101.8726) (64.6884, 101.8622) knots 0 0 0 1 2 3 4 5 6 6 6
  line L409 (64.6884, 101.8622) -> (64.6261, 102.1968)
  spline S346 degree 2 poles (64.6261, 102.1968) (64.8673, 102.2098) (65.2901, 102.4147) (65.6117, 102.7518) (65.8114, 103.2057) (65.8244, 103.4625) knots 0 0 0 1 2 3 4 4 4
  line L410 (65.8244, 103.4625) -> (65.6636, 103.2264)
  spline S347 degree 2 poles (65.801, 103.8074) (65.7958, 103.9578) (65.718, 104.2405) (65.578, 104.4636) (65.3627, 104.5984) (65.2201, 104.5984) knots 0 0 0 1 2 3 4 4 4
  spline S348 degree 2 poles (65.2201, 104.5984) (65.0826, 104.5984) (64.8673, 104.5102) (64.7143, 104.3546) (64.6313, 104.1342) (64.6313, 104.0019) knots 0 0 0 1 2 3 4 4 4
  spline S349 degree 2 poles (64.6313, 104.0019) (64.6313, 103.8696) (64.6988, 103.6466) (64.831, 103.4806) (65.0385, 103.3872) (65.176, 103.3872) knots 0 0 0 1 2 3 4 4 4
  spline S350 degree 2 poles (65.176, 103.3872) (65.2823, 103.3872) (65.4768, 103.4547) (65.6402, 103.5688) (65.7647, 103.7218) (65.801, 103.8074) knots 0 0 0 1 2 3 4 4 4
  line L411 (67.2223, 104.9071) -> (67.2223, 104.7074)
  spline S351 degree 2 poles (67.2223, 104.7074) (67.2223, 104.6295) (67.1937, 104.4065) (67.1782, 104.2976) knots 0 0 0 1 2 2 2
  spline S352 degree 2 poles (67.1782, 104.2976) (67.1574, 104.1731) (67.1341, 104.0382) knots 0 0 0 1 1 1
  line L412 (67.1341, 104.0382) -> (66.9603, 104.0382)
  spline S353 degree 2 poles (66.9603, 104.0382) (66.937, 104.1731) (66.9162, 104.2976) knots 0 0 0 1 1 1
  spline S354 degree 2 poles (66.9162, 104.2976) (66.9007, 104.4065) (66.8721, 104.6295) (66.8721, 104.7074) knots 0 0 0 1 2 2 2
  line L413 (66.8721, 104.7074) -> (66.8721, 104.9071)
  line L414 (66.8721, 104.9071) -> (67.2223, 104.9071)
  line L415 (67.8266, 104.9071) -> (67.8266, 104.7074)
  spline S355 degree 2 poles (67.8266, 104.7074) (67.8266, 104.6295) (67.798, 104.4065) (67.7825, 104.2976) knots 0 0 0 1 2 2 2
  spline S356 degree 2 poles (67.7825, 104.2976) (67.7617, 104.1731) (67.7384, 104.0382) knots 0 0 0 1 1 1
  line L416 (67.7384, 104.0382) -> (67.5646, 104.0382)
  spline S357 degree 2 poles (67.5646, 104.0382) (67.5413, 104.1731) (67.5205, 104.2976) knots 0 0 0 1 1 1
  spline S358 degree 2 poles (67.5205, 104.2976) (67.505, 104.4065) (67.4764, 104.6295) (67.4764, 104.7074) knots 0 0 0 1 2 2 2
  line L417 (67.4764, 104.7074) -> (67.4764, 104.9071)
  line L418 (67.4764, 104.9071) -> (67.8266, 104.9071)
  spline S359 degree 2 poles (70.3656, 102.6507) (70.3656, 102.5184) (70.3968, 102.3395) (70.4538, 102.2305) (70.5394, 102.1838) (70.5965, 102.1838) knots 0 0 0 1 2 3 4 4 4
  spline S360 degree 2 poles (70.5965, 102.1838) (70.6406, 102.1838) (70.7132, 102.1942) (70.7391, 102.202) knots 0 0 0 1 2 2 2
  spline S361 degree 2 poles (70.7391, 102.202) (70.7702, 102.2098) (70.7936, 102.2202) knots 0 0 0 1 1 1
  line L419 (70.7936, 102.2202) -> (70.931, 101.9764)
  spline S362 degree 2 poles (70.931, 101.9764) (70.9155, 101.9608) (70.8454, 101.9219) (70.7495, 101.8856) (70.6276, 101.8622) (70.5576, 101.8622) knots 0 0 0 1 2 3 4 4 4
  spline S363 degree 2 poles (70.5576, 101.8622) (70.376, 101.8622) (70.1504, 101.9945) (70.0259, 102.2227) (69.9844, 102.5262) (69.9844, 102.6974) knots 0 0 0 1 2 3 4 4 4
  line L420 (69.9844, 102.6974) -> (69.9844, 103.7815)
  line L421 (69.9844, 103.7815) -> (69.6835, 103.7815)
  line L422 (69.6835, 103.7815) -> (69.6835, 104.1031)
  line L423 (69.6835, 104.1031) -> (69.9844, 104.1031)
  line L424 (69.9844, 104.1031) -> (69.9844, 104.5232)
  line L425 (69.9844, 104.5232) -> (70.3553, 104.7463)
  line L426 (70.3553, 104.7463) -> (70.3553, 104.1031)
  line L427 (70.3553, 104.1031) -> (71.0374, 104.1031)
  line L428 (71.0374, 104.1031) -> (70.9985, 103.7815)
  line L429 (70.9985, 103.7815) -> (70.3656, 103.7815)
  line L430 (70.3656, 103.7815) -> (70.3656, 102.6507)
  spline S364 degree 2 poles (73.1252, 102.1553) (73.0629, 102.0905) (72.9151, 101.9841) (72.7335, 101.9037) (72.5157, 101.8622) (72.3808, 101.8622) knots 0 0 0 1 2 3 4 4 4
  spline S365 degree 2 poles (72.3808, 101.8622) (72.1137, 101.8622) (71.7376, 102.0516) (71.499, 102.368) (71.3875, 102.7778) (71.3875, 103.0008) knots 0 0 0 1 2 3 4 4 4
  spline S366 degree 2 poles (71.3875, 103.0008) (71.3875, 103.1435) (71.4394, 103.4236) (71.5431, 103.6751) (71.7013, 103.893) (71.9088, 104.0486) (72.1733, 104.1394) (72.3315, 104.1394) knots 0 0 0 1 2 3 4 5 6 6 6
  spline S367 degree 2 poles (72.3315, 104.1394) (72.5468, 104.1394) (72.8658, 103.9993) (73.0733, 103.7452) (73.1744, 103.3924) (73.1744, 103.1772) knots 0 0 0 1 2 3 4 4 4
  spline S368 degree 2 poles (73.1744, 103.1772) (73.1744, 103.1149) (73.1667, 102.9671) (73.1589, 102.8997) knots 0 0 0 1 2 2 2
  line L431 (73.1589, 102.8997) -> (71.7687, 102.8997)
  spline S369 degree 2 poles (71.7687, 102.8997) (71.7687, 102.7492) (71.8517, 102.4899) (71.9996, 102.2954) (72.2096, 102.1838) (72.3419, 102.1838) knots 0 0 0 1 2 3 4 4 4
  spline S370 degree 2 poles (72.3419, 102.1838) (72.469, 102.1838) (72.6609, 102.2227) (72.7958, 102.2772) (72.884, 102.3317) (72.9073, 102.3472) knots 0 0 0 1 2 3 4 4 4
  line L432 (72.9073, 102.3472) -> (73.1252, 102.1553)
  spline S371 degree 2 poles (72.7932, 103.2005) (72.7958, 103.2239) (72.7984, 103.2679) (72.7984, 103.2887) knots 0 0 0 1 2 2 2
  spline S372 degree 2 poles (72.7984, 103.2887) (72.7984, 103.4028) (72.7439, 103.5973) (72.6376, 103.74) (72.4742, 103.8204) (72.3601, 103.8204) knots 0 0 0 1 2 3 4 4 4
  spline S373 degree 2 poles (72.3601, 103.8204) (72.2278, 103.8204) (72.0359, 103.7348) (71.9062, 103.5999) (71.8258, 103.4391) (71.8076, 103.3665) knots 0 0 0 1 2 3 4 4 4
  line L433 (71.8076, 103.3665) -> (71.7013, 103.146)
  line L434 (71.7013, 103.146) -> (72.0592, 103.2005)
  line L435 (72.0592, 103.2005) -> (72.7932, 103.2005)
  line L436 (74.1781, 101.896) -> (73.7969, 101.896)
  line L437 (73.7969, 101.896) -> (73.7969, 104.1057)
  line L438 (73.7969, 104.1057) -> (74.1781, 104.1446)
  line L439 (74.1781, 104.1446) -> (74.1781, 103.7763)
  line L440 (74.1781, 103.7763) -> (74.3, 103.9915)
  spline S374 degree 2 poles (74.3, 103.9915) (74.3363, 104.0175) (74.4453, 104.0693) (74.5827, 104.1108) (74.7383, 104.1394) (74.8213, 104.1394) knots 0 0 0 1 2 3 4 4 4
  spline S375 degree 2 poles (74.8213, 104.1394) (75.0444, 104.1394) (75.3271, 103.9189) (75.3686, 103.7503) knots 0 0 0 1 2 2 2
  line L441 (75.3686, 103.7503) -> (75.5216, 103.9838)
  spline S376 degree 2 poles (75.5216, 103.9838) (75.5916, 104.0408) (75.8484, 104.1394) (76.0144, 104.1394) knots 0 0 0 1 2 2 2
  spline S377 degree 2 poles (76.0144, 104.1394) (76.1674, 104.1394) (76.3852, 104.0382) (76.5227, 103.8437) (76.5875, 103.5714) (76.5875, 103.4028) knots 0 0 0 1 2 3 4 4 4
  line L442 (76.5875, 103.4028) -> (76.5875, 101.896)
  line L443 (76.5875, 101.896) -> (76.2063, 101.896)
  line L444 (76.2063, 101.896) -> (76.2063, 103.3821)
  spline S378 degree 2 poles (76.2063, 103.3821) (76.2063, 103.491) (76.1752, 103.6544) (76.1025, 103.7633) (75.9781, 103.8178) (75.8847, 103.8178) knots 0 0 0 1 2 3 4 4 4
  spline S379 degree 2 poles (75.8847, 103.8178) (75.8276, 103.8178) (75.7005, 103.7789) (75.5709, 103.7114) (75.449, 103.6258) (75.3945, 103.5818) knots 0 0 0 1 2 3 4 4 4
  spline S380 degree 2 poles (75.3945, 103.5818) (75.3997, 103.5221) (75.4023, 103.4443) (75.4023, 103.3821) knots 0 0 0 1 2 2 2
  line L445 (75.4023, 103.3821) -> (75.4023, 101.896)
  line L446 (75.4023, 101.896) -> (75.021, 101.896)
  line L447 (75.021, 101.896) -> (75.021, 103.3821)
  spline S381 degree 2 poles (75.021, 103.3821) (75.021, 103.5999) (74.8758, 103.8178) (74.6891, 103.8178) knots 0 0 0 1 2 2 2
  spline S382 degree 2 poles (74.6891, 103.8178) (74.6294, 103.8178) (74.492, 103.7815) (74.3597, 103.7166) (74.23, 103.6362) (74.1781, 103.5921) knots 0 0 0 1 2 3 4 4 4
  line L448 (74.1781, 103.5921) -> (74.1781, 101.896)
  line L449 (77.4097, 100.8923) -> (77.4097, 104.1057)
  line L450 (77.4097, 104.1057) -> (77.7909, 104.1446)
  line L451 (77.7909, 104.1446) -> (77.7909, 103.7918)
  line L452 (77.7909, 103.7918) -> (77.9803, 104.046)
  spline S383 degree 2 poles (77.9803, 104.046) (78.0399, 104.0823) (78.2552, 104.1394) (78.4108, 104.1394) knots 0 0 0 1 2 2 2
  spline S384 degree 2 poles (78.4108, 104.1394) (78.5768, 104.1394) (78.8698, 103.9838) (79.0877, 103.6933) (79.2148, 103.2835) (79.2148, 103.0319) knots 0 0 0 1 2 3 4 4 4
  spline S385 degree 2 poles (79.2148, 103.0319) (79.2148, 102.7829) (79.054, 102.368) (78.7583, 102.0645) (78.3408, 101.896) (78.0814, 101.896) knots 0 0 0 1 2 3 4 4 4
  line L453 (78.0814, 101.896) -> (77.7909, 101.896)
  line L454 (77.7909, 101.896) -> (77.7909, 100.8923)
  line L455 (77.7909, 100.8923) -> (77.4097, 100.8923)
  line L456 (77.7909, 102.2176) -> (78.1203, 102.2176)
  spline S386 degree 2 poles (78.1203, 102.2176) (78.3045, 102.2176) (78.5742, 102.3395) (78.7505, 102.5599) (78.8335, 102.8711) (78.8335, 103.0579) knots 0 0 0 1 2 3 4 4 4
  spline S387 degree 2 poles (78.8335, 103.0579) (78.8335, 103.2524) (78.7583, 103.5403) (78.6261, 103.727) (78.4497, 103.8178) (78.3511, 103.8178) knots 0 0 0 1 2 3 4 4 4
  spline S388 degree 2 poles (78.3511, 103.8178) (78.2552, 103.8178) (78.084, 103.7685) (77.9414, 103.6907) (77.8298, 103.5999) (77.7909, 103.5558) knots 0 0 0 1 2 3 4 4 4
  line L457 (77.7909, 103.5558) -> (77.7909, 102.2176)
  spline S389 degree 2 poles (80.2003, 102.6507) (80.2003, 102.5184) (80.2315, 102.3395) (80.2885, 102.2305) (80.3741, 102.1838) (80.4312, 102.1838) knots 0 0 0 1 2 3 4 4 4
  spline S390 degree 2 poles (80.4312, 102.1838) (80.4752, 102.1838) (80.5479, 102.1942) (80.5738, 102.202) knots 0 0 0 1 2 2 2
  spline S391 degree 2 poles (80.5738, 102.202) (80.6049, 102.2098) (80.6283, 102.2202) knots 0 0 0 1 1 1
  line L458 (80.6283, 102.2202) -> (80.7657, 101.9764)
  spline S392 degree 2 poles (80.7657, 101.9764) (80.7502, 101.9608) (80.6801, 101.9219) (80.5842, 101.8856) (80.4623, 101.8622) (80.3923, 101.8622) knots 0 0 0 1 2 3 4 4 4
  spline S393 degree 2 poles (80.3923, 101.8622) (80.2107, 101.8622) (79.9851, 101.9945) (79.8606, 102.2227) (79.8191, 102.5262) (79.8191, 102.7) knots 0 0 0 1 2 3 4 4 4
  line L459 (79.8191, 102.7) -> (79.8191, 104.7074)
  line L460 (79.8191, 104.7074) -> (79.7802, 105.1094)
  line L461 (79.7802, 105.1094) -> (80.2003, 105.1483)
  line L462 (80.2003, 105.1483) -> (80.2003, 102.6507)
  line L463 (82.6694, 101.896) -> (82.2492, 101.896)
  line L464 (82.2492, 101.896) -> (82.2492, 102.2202)
  line L465 (82.2492, 102.2202) -> (82.0599, 101.9971)
  spline S394 degree 2 poles (82.0599, 101.9971) (82.0262, 101.9712) (81.938, 101.9219) (81.8472, 101.883) (81.7565, 101.8622) (81.7176, 101.8622) knots 0 0 0 1 2 3 4 4 4
  spline S395 degree 2 poles (81.7176, 101.8622) (81.5671, 101.8622) (81.2922, 101.9556) (81.0847, 102.1398) (80.9628, 102.4095) (80.9628, 102.5884) knots 0 0 0 1 2 3 4 4 4
  spline S396 degree 2 poles (80.9628, 102.5884) (80.9628, 102.7752) (81.1133, 103.0501) (81.3493, 103.2316) (81.6372, 103.3224) (81.7772, 103.3224) knots 0 0 0 1 2 3 4 4 4
  spline S397 degree 2 poles (81.7772, 103.3224) (81.8913, 103.3224) (82.0651, 103.2991) (82.1273, 103.2835) knots 0 0 0 1 2 2 2
  spline S398 degree 2 poles (82.1273, 103.2835) (82.1974, 103.2653) (82.2492, 103.242) knots 0 0 0 1 1 1
  line L466 (82.2492, 103.242) -> (82.2492, 103.312)
  spline S399 degree 2 poles (82.2492, 103.312) (82.2492, 103.4313) (82.2207, 103.6181) (82.1351, 103.7503) (81.9717, 103.8178) (81.8369, 103.8178) knots 0 0 0 1 2 3 4 4 4
  spline S400 degree 2 poles (81.8369, 103.8178) (81.7279, 103.8178) (81.5282, 103.7866) (81.4504, 103.7685) knots 0 0 0 1 2 2 2
  spline S401 degree 2 poles (81.4504, 103.7685) (81.357, 103.7477) (81.2792, 103.7244) knots 0 0 0 1 1 1
  line L467 (81.2792, 103.7244) -> (81.134, 103.9915)
  spline S402 degree 2 poles (81.134, 103.9915) (81.2222, 104.033) (81.3337, 104.0642) knots 0 0 0 1 1 1
  spline S403 degree 2 poles (81.3337, 104.0642) (81.4297, 104.0927) (81.6968, 104.1394) (81.8576, 104.1394) knots 0 0 0 1 2 2 2
  spline S404 degree 2 poles (81.8576, 104.1394) (82.0884, 104.1394) (82.3893, 104.0149) (82.563, 103.7892) (82.6305, 103.4754) (82.6305, 103.2809) knots 0 0 0 1 2 3 4 4 4
  line L468 (82.6305, 103.2809) -> (82.6305, 102.2565)
  line L469 (82.6305, 102.2565) -> (82.6694, 101.896)
  spline S405 degree 2 poles (82.2492, 102.9671) (82.1922, 102.9749) (82.1273, 102.9827) knots 0 0 0 1 1 1
  spline S406 degree 2 poles (82.1273, 102.9827) (82.0755, 102.9878) (81.9328, 103.0008) (81.8576, 103.0008) knots 0 0 0 1 2 2 2
  spline S407 degree 2 poles (81.8576, 103.0008) (81.7435, 103.0008) (81.5568, 102.9567) (81.4193, 102.8582) (81.3441, 102.7026) (81.3441, 102.5884) knots 0 0 0 1 2 3 4 4 4
  spline S408 degree 2 poles (81.3441, 102.5884) (81.3441, 102.5003) (81.4037, 102.3498) (81.5101, 102.2409) (81.6527, 102.1838) (81.7331, 102.1838) knots 0 0 0 1 2 3 4 4 4
  spline S409 degree 2 poles (81.7331, 102.1838) (81.772, 102.1838) (81.8602, 102.2072) (81.9458, 102.2409) (82.0314, 102.2902) (82.0703, 102.3135) knots 0 0 0 1 2 3 4 4 4
  spline S410 degree 2 poles (82.0703, 102.3135) (82.161, 102.3732) (82.2492, 102.4458) knots 0 0 0 1 1 1
  line L470 (82.2492, 102.4458) -> (82.2492, 102.9671)
  spline S411 degree 2 poles (83.7146, 102.6507) (83.7146, 102.5184) (83.7457, 102.3395) (83.8028, 102.2305) (83.8883, 102.1838) (83.9454, 102.1838) knots 0 0 0 1 2 3 4 4 4
  spline S412 degree 2 poles (83.9454, 102.1838) (83.9895, 102.1838) (84.0621, 102.1942) (84.088, 102.202) knots 0 0 0 1 2 2 2
  spline S413 degree 2 poles (84.088, 102.202) (84.1192, 102.2098) (84.1425, 102.2202) knots 0 0 0 1 1 1
  line L471 (84.1425, 102.2202) -> (84.28, 101.9764)
  spline S414 degree 2 poles (84.28, 101.9764) (84.2644, 101.9608) (84.1944, 101.9219) (84.0984, 101.8856) (83.9765, 101.8622) (83.9065, 101.8622) knots 0 0 0 1 2 3 4 4 4
  spline S415 degree 2 poles (83.9065, 101.8622) (83.7249, 101.8622) (83.4993, 101.9945) (83.3748, 102.2227) (83.3333, 102.5262) (83.3333, 102.6974) knots 0 0 0 1 2 3 4 4 4
  line L472 (83.3333, 102.6974) -> (83.3333, 103.7815)
  line L473 (83.3333, 103.7815) -> (83.0325, 103.7815)
  line L474 (83.0325, 103.7815) -> (83.0325, 104.1031)
  line L475 (83.0325, 104.1031) -> (83.3333, 104.1031)
  line L476 (83.3333, 104.1031) -> (83.3333, 104.5232)
  line L477 (83.3333, 104.5232) -> (83.7042, 104.7463)
  line L478 (83.7042, 104.7463) -> (83.7042, 104.1031)
  line L479 (83.7042, 104.1031) -> (84.3863, 104.1031)
  line L480 (84.3863, 104.1031) -> (84.3474, 103.7815)
  line L481 (84.3474, 103.7815) -> (83.7146, 103.7815)
  line L482 (83.7146, 103.7815) -> (83.7146, 102.6507)
  spline S416 degree 2 poles (86.4741, 102.1553) (86.4119, 102.0905) (86.264, 101.9841) (86.0825, 101.9037) (85.8646, 101.8622) (85.7298, 101.8622) knots 0 0 0 1 2 3 4 4 4
  spline S417 degree 2 poles (85.7298, 101.8622) (85.4626, 101.8622) (85.0866, 102.0516) (84.848, 102.368) (84.7364, 102.7778) (84.7364, 103.0008) knots 0 0 0 1 2 3 4 4 4
  spline S418 degree 2 poles (84.7364, 103.0008) (84.7364, 103.1435) (84.7883, 103.4236) (84.892, 103.6751) (85.0502, 103.893) (85.2577, 104.0486) (85.5223, 104.1394) (85.6805, 104.1394) knots 0 0 0 1 2 3 4 5 6 6 6
  spline S419 degree 2 poles (85.6805, 104.1394) (85.8957, 104.1394) (86.2147, 103.9993) (86.4222, 103.7452) (86.5234, 103.3924) (86.5234, 103.1772) knots 0 0 0 1 2 3 4 4 4
  spline S420 degree 2 poles (86.5234, 103.1772) (86.5234, 103.1149) (86.5156, 102.9671) (86.5078, 102.8997) knots 0 0 0 1 2 2 2
  line L483 (86.5078, 102.8997) -> (85.1177, 102.8997)
  spline S421 degree 2 poles (85.1177, 102.8997) (85.1177, 102.7492) (85.2007, 102.4899) (85.3485, 102.2954) (85.5586, 102.1838) (85.6909, 102.1838) knots 0 0 0 1 2 3 4 4 4
  spline S422 degree 2 poles (85.6909, 102.1838) (85.8179, 102.1838) (86.0099, 102.2227) (86.1447, 102.2772) (86.2329, 102.3317) (86.2562, 102.3472) knots 0 0 0 1 2 3 4 4 4
  line L484 (86.2562, 102.3472) -> (86.4741, 102.1553)
  spline S423 degree 2 poles (86.1421, 103.2005) (86.1447, 103.2239) (86.1473, 103.2679) (86.1473, 103.2887) knots 0 0 0 1 2 2 2
  spline S424 degree 2 poles (86.1473, 103.2887) (86.1473, 103.4028) (86.0928, 103.5973) (85.9865, 103.74) (85.8231, 103.8204) (85.709, 103.8204) knots 0 0 0 1 2 3 4 4 4
  spline S425 degree 2 poles (85.709, 103.8204) (85.5767, 103.8204) (85.3848, 103.7348) (85.2551, 103.5999) (85.1747, 103.4391) (85.1566, 103.3665) knots 0 0 0 1 2 3 4 4 4
  line L485 (85.1566, 103.3665) -> (85.0502, 103.146)
  line L486 (85.0502, 103.146) -> (85.4082, 103.2005)
  line L487 (85.4082, 103.2005) -> (86.1421, 103.2005)
  line L488 (89.7757, 102.1683) -> (89.6019, 101.9478)
  spline S426 degree 2 poles (89.6019, 101.9478) (89.5838, 101.9349) (89.5163, 101.9063) (89.4204, 101.8804) (89.2907, 101.8622) (89.2129, 101.8622) knots 0 0 0 1 2 3 4 4 4
  spline S427 degree 2 poles (89.2129, 101.8622) (89.0313, 101.8622) (88.7149, 102.0412) (88.4815, 102.3472) (88.3492, 102.7596) (88.3492, 102.9904) knots 0 0 0 1 2 3 4 4 4